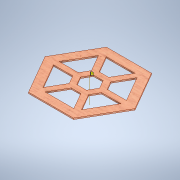
# Autodesk Inventor part: LightFrontalino
Saved by Autodesk Inventor 2020 (Build 240168000, 168)
## iProperties
Created: 2020-04-08
Part Number: LightFrontalino
Material: Wood (Oak)
Document SubType Name: Modeling
Designer: Samuele
Density: 0.76 g/cm^3
Appearance: White Oak - Natural Medium Gloss
Author: Samuele
Autodesk Inventor part; units mm, degrees
ref_plane "YZ Plane" through (0, 0, 0) normal (1, 0, 0) x (0, 1, 0)
ref_plane "XZ Plane" through (0, 0, 0) normal (0, 1, 0) x (-1, 0, 0)
ref_plane "XY Plane" through (0, 0, 0) normal (0, 0, 1) x (1, 0, 0)
sketch "Sketch6" plane through (0, 0, 0) normal (0, 1, 0) x (-1, 0, 0)
  circle A0 centre (32.5, -48.5) radius 70
  line L0 (102.5, -48.5) -> (67.5, -109.1218)
  line L1 (67.5, -109.1218) -> (-2.5, -109.1218)
  line L2 (-2.5, -109.1218) -> (-37.5, -48.5)
  line L3 (-37.5, -48.5) -> (-2.5, 12.1218)
  line L4 (-2.5, 12.1218) -> (67.5, 12.1218)
  line L5 (67.5, 12.1218) -> (102.5, -48.5)
  line L6 (32.5, 12.1218) -> (47.5, 12.1218)
  line L7 (47.5, 12.1218) -> (47.5, 5.6218)
  line L8 (47.5, 5.6218) -> (17.5, 5.6218)
  line L9 (17.5, 5.6218) -> (17.5, 12.1218)
  line L10 (47.5, 5.6218) -> (56.6924, 5.6218) construction
  line L11 (17.5, 8.8718) -> (20, 8.8718)
  line L12 (47.5, 8.8718) -> (45, 8.8718)
  line L13 (45, 8.8718) -> (45, 10.1218)
  line L14 (45, 10.1218) -> (20, 10.1218)
  line L15 (20, 10.1218) -> (20, 7.6218)
  line L16 (20, 7.6218) -> (45, 7.6218)
  line L17 (45, 7.6218) -> (45, 10.1218)
  line L18 (47.5, 5.6218) -> (56.6924, 5.6218)
  line L19 (17.5, 5.6218) -> (11, 5.6218)
  line L20 (17.5, 12.1218) -> (11, 5.6218)
  line L21 (17.5, 12.1218) -> (26.6924, 12.1218) construction
  line L22 (47.5, 12.1218) -> (54, 5.6218)
  line L23 (85, -18.1891) -> (77.5, -5.1987)
  line L24 (77.5, -5.1987) -> (71.8708, -8.4487)
  line L25 (71.8708, -8.4487) -> (86.8708, -34.4295)
  line L26 (86.8708, -34.4295) -> (92.5, -31.1795)
  line L27 (71.8708, -8.4487) -> (67.2746, -0.4879) construction
  line L28 (89.6854, -32.8045) -> (88.4354, -30.6394)
  line L29 (74.6854, -6.8237) -> (75.9354, -8.9888)
  line L30 (75.9354, -8.9888) -> (77.0179, -8.3638)
  line L31 (77.0179, -8.3638) -> (89.5179, -30.0144)
  line L32 (89.5179, -30.0144) -> (87.3529, -31.2644)
  line L33 (87.3529, -31.2644) -> (74.8529, -9.6138)
  line L34 (74.8529, -9.6138) -> (77.0179, -8.3638)
  line L35 (71.8708, -8.4487) -> (67.2746, -0.4879)
  line L36 (86.8708, -34.4295) -> (90.1208, -40.0587)
  line L37 (92.5, -31.1795) -> (90.1208, -40.0587)
  line L38 (92.5, -31.1795) -> (87.9038, -23.2187) construction
  line L39 (77.5, -5.1987) -> (68.6208, -2.8196)
  line L40 (71.8708, -88.5513) -> (67.2746, -96.5121) construction
  line L41 (74.6854, -90.1763) -> (75.9354, -88.0112)
  line L42 (74.8529, -87.3862) -> (77.0179, -88.6362)
  line L43 (77.5, -91.8013) -> (71.8708, -88.5513)
  line L44 (77.5, -91.8013) -> (68.6208, -94.1804)
  line L45 (71.8708, -88.5513) -> (67.2746, -96.5121)
  line L46 (77.0179, -88.6362) -> (89.5179, -66.9856)
  line L47 (87.3529, -65.7356) -> (74.8529, -87.3862)
  line L48 (71.8708, -88.5513) -> (86.8708, -62.5705)
  line L49 (89.5179, -66.9856) -> (87.3529, -65.7356)
  line L50 (89.6854, -64.1955) -> (88.4354, -66.3606)
  line L51 (86.8708, -62.5705) -> (92.5, -65.8205)
  line L52 (86.8708, -62.5705) -> (90.1208, -56.9413)
  line L53 (92.5, -65.8205) -> (90.1208, -56.9413)
  line L54 (94.9944, -48.5) -> (63.7472, -102.6218)
  line L55 (63.7472, -102.6218) -> (1.2528, -102.6218)
  line L56 (1.2528, -102.6218) -> (-29.9944, -48.5)
  line L57 (-29.9944, -48.5) -> (1.2528, 5.6218)
  line L58 (1.2528, 5.6218) -> (63.7472, 5.6218)
  line L59 (63.7472, 5.6218) -> (94.9944, -48.5)
  line L60 (74.8529, -87.3862) -> (73.1208, -86.3862)
  line L61 (87.3529, -65.7356) -> (85.6208, -64.7356)
  line L62 (87.3529, -31.2644) -> (85.6208, -32.2644)
  line L63 (74.8529, -9.6138) -> (73.1208, -10.6138)
  line L64 (45, 7.6218) -> (45, 5.6218)
  line L65 (20, 7.6218) -> (20, 5.6218)
  line L66 (-29.9944, -48.5) -> (-22.9944, -48.5)
  line L67 (-29.9944, -48.5) -> (-28.2944, -48.5)
  line L68 (-28.2944, -48.5) -> (-22.9944, -48.5)
  circle A1 centre (-26.9944, -48.5) radius 1.5
  line L69 (-29.9944, -48.5) -> (-23.9944, -48.5)
  line L70 (-23.9944, -48.5) -> (-26.9944, -53.6962)
  line L71 (-23.9944, -48.5) -> (-26.9944, -43.3038)
  point P0 (-27.5473, -52.7386)
  point P1 (-28.2775, -45.5261)
  point P2 (88.4354, -30.6394)
  point P3 (75.9354, -8.9888)
  point P4 (76.4767, -8.6763)
  point P5 (89.6854, -32.8045)
  point P6 (86.4869, -65.2356)
  point P7 (88.4354, -66.3606)
  dimension "d127" = 140
  dimension "d87" = 15
  dimension "d88" = 6.5
  dimension "d91" = 2.5
  dimension "d92" = 2.5
  dimension "d95" = 1.25
  dimension "d96" = 25
  dimension "d97" = 2.5
  dimension "d98" = 25
  dimension "d99" = 135
  dimension "d100" = 0
  dimension "d114" = 1.7
  dimension "d117" = 3
  dimension "d121" = 3
  dimension "d123" = 6
  dimension "d128" = 5.1962
  dimension "d129" = 5.1962
  dimension "d130" = 3
  constraints: 144 end point, 17 point on line, 9 midpoint, 8 perpendicular, 6 horizontal, 3 vertical, 2 collinear, 2 horizontal alignment, 2 parallel, 1 centre point, 1 equal length, 49 other
  measures "d87" distance of L6.start L6.end
  measures "d88" distance of L6.end L7.end
  measures "d91" distance of L11.start L11.end
  measures "d92" distance of L12.start L12.end
  measures "d95" distance of L12.end L13.end
  measures "d96" distance of L13.end L14.end
  measures "d97" distance of L14.end L15.end
  measures "d98" distance of L15.end L16.end
  measures "d99" angle of L20 L21
  measures "d100" distance of L9.end L20.start
  measures "d114" distance of L56.end L67.end
  measures "d117" diameter of A1
  measures "d121" distance of L56.end A1.centre
  measures "d123" distance of L56.end L69.end
  measures "d128" vertical distance of L69.end L70.end
  measures "d129" vertical distance of L69.end L71.end
  measures "d130" distance of L69.end A1.centre
extrude "Fronte" add sketch "Sketch6" along normal blind 2 contours L0 L53 L54 L59 L37 L5 | L5 L39 L35 L59 L58 L18 L22 L4 | L1 L2 L3 L4 L20 L58 L57 L56 L55 L54 L45 L44 L0 | L0 L43 L41 L42 L46 L49 L50 L51 | L51 L52 L53 | L26 L28 L32 L31 L30 L29 L24 L5 | L37 L36 L26 | L7 L12 L13 L14 L15 L11 L9 L4 | L22 L18 L7 | L24 L35 L39 | L44 L45 L43 | L50 L49 L61 L48 L51 | L52 L48 L45 L54 L55 L56 L70 L71 L57 L58 L19 L8 L18 L59 L35 L25 L36 | L26 L25 L62 L32 L28 | L9 L19 L20 | L7 L8 L64 L17 L12 | L29 L34 L63 L25 L24 | L43 L48 L60 L42 L41 | L49 L46 L42 L47 | L32 L33 L34 L30 L31 | L11 L15 L65 L8 L9 | L17 L16 L15 L14 L13 | L47 L60 L48 L61 | L25 L63 L33 L62 | L8 L65 L16 L64 | L71 L66 A1 L57 | L66 A1 L70 L56 | A1 L66 | L66 A1
sketch "Sketch11" plane through (0, 0, 0) normal (0, -1, 0) x (1, 0, 0)
  line L0 (-63.7472, 5.6218) -> (-1.2528, -102.6218)
  line L1 (-94.9944, -48.5) -> (29.9944, -48.5)
  line L2 (-63.7472, -102.6218) -> (-1.2528, 5.6218)
  line L3 (-1.2528, 5.6218) -> (-1.2528, -102.6218)
  circle A0 centre (-32.5, -48.5) radius 55
  line L4 (-5, -0.8686) -> (22.5, -48.5)
  line L5 (22.5, -48.5) -> (-5, -96.1314)
  line L6 (-5, -96.1314) -> (-60, -96.1314)
  line L7 (-60, -96.1314) -> (-87.5, -48.5)
  line L8 (-87.5, -48.5) -> (-60, -0.8686)
  line L9 (-60, -0.8686) -> (-5, -0.8686)
  circle A1 centre (-32.5, -48.5) radius 25
  circle A2 centre (-32.5, -48.5) radius 15
  line L10 (-25, -35.5096) -> (-17.5, -48.5)
  line L11 (-17.5, -48.5) -> (-25, -61.4904)
  line L12 (-25, -61.4904) -> (-40, -61.4904)
  line L13 (-40, -61.4904) -> (-47.5, -48.5)
  line L14 (-47.5, -48.5) -> (-40, -35.5096)
  line L15 (-40, -35.5096) -> (-25, -35.5096)
  line L16 (-20, -26.8494) -> (-7.5, -48.5)
  line L17 (-7.5, -48.5) -> (-20, -70.1506)
  line L18 (-20, -70.1506) -> (-45, -70.1506)
  line L19 (-45, -70.1506) -> (-57.5, -48.5)
  line L20 (-57.5, -48.5) -> (-45, -26.8494)
  line L21 (-45, -26.8494) -> (-20, -26.8494)
  line L22 (-85, -44.1699) -> (-55, -44.1699)
  line L23 (-85, -52.8301) -> (-55, -52.8301)
  line L24 (-55, -96.1314) -> (-40, -70.1506)
  line L25 (-62.5, -91.8013) -> (-47.5, -65.8205)
  line L26 (-2.5, -91.8013) -> (-17.5, -65.8205)
  line L27 (-10, -96.1314) -> (-25, -70.1506)
  line L28 (20, -44.1699) -> (-10, -44.1699)
  line L29 (20, -52.8301) -> (-10, -52.8301)
  line L30 (-10, -0.8686) -> (-25, -26.8494)
  line L31 (-2.5, -5.1987) -> (-17.5, -31.1795)
  line L32 (-62.5, -5.1987) -> (-47.5, -31.1795)
  line L33 (-55, -0.8686) -> (-40, -26.8494)
  line L34 (-43.75, -42.0048) -> (-51.25, -37.6747)
  line L35 (-70, -52.8301) -> (-70, -44.1699)
  point P0 (0, 0)
  point P1 (-62.5, -91.8013)
  point P2 (-47.5, -65.8205)
  point P3 (-10, -96.1314)
  point P4 (-25, -70.1506)
  point P5 (-55, -96.1314)
  point P6 (-10, -52.8301)
  point P7 (-2.5, -91.8013)
  point P8 (20, -52.8301)
  point P9 (20, -44.1699)
  point P10 (-2.5, -5.1987)
  point P11 (-17.5, -31.1795)
  point P12 (-10, -44.1699)
  point P13 (-62.5, -5.1987)
  point P14 (-47.5, -31.1795)
  point P15 (-55, -0.8686)
  point P16 (-40, -26.8494)
  point P17 (-25, -26.8494)
  point P18 (-10, -0.8686)
  dimension "d158" = 110
  dimension "d159" = 50
  dimension "d160" = 30
  dimension "d164" = 360
  constraints: 72 end point, 7 point on line, 6 coincident, 5 midpoint, 1 equal length, 1 parallel, 1 perpendicular, 88 other
extrude "Extrusion17" cut sketch "Sketch11" against normal blind 2 contours L32 A1 L22 L8 | L9 L30 A1 L33 | L15 L2 L0 | L0 L1 L14 | A1 L30 L21 L33 | L32 L20 L22 A1 | L4 L3 L28 A1 L31 | L23 A1 L25 L7 | L1 L11 L0 | L2 L13 L1 | L2 L10 L1 | L0 L12 L2 | A1 L28 L16 L31 | L4 L28 L3 | L24 A1 L27 L6 | L5 L3 L29 | L23 L19 L25 A1 | L24 L18 L27 A1 | L26 A1 L29 L3 L5 | L26 L17 L29 A1
body "Solid3"
